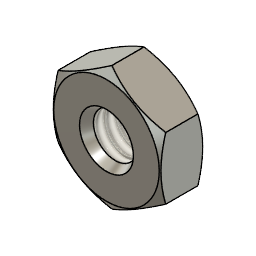
Gimbal Mechanism - Model Rocketry (Autodesk Fusion 360 archive; units mm, degrees)
design "Hexagon Regular Nut ISO 4032 - M2 Steel 6 Plain"
description: Hexagon Regular Nut ISO 4032 - M2
part number: ISO 4032 - M2 Steel 6 Plain
Autodesk Fusion 360 part; units mm, degrees
sketch "Sketch1" plane through (0, 0, 0) normal (0, 1, 0) x (1, 0, 0)
  line L0 (0, 0) -> (0, -1.6)
  line L1 (-1, 0) -> (-1.96, 0)
  line L2 (-1.96, 0) -> (-2.31, -0.2021)
  line L3 (-2.31, -0.2021) -> (-2.31, -1.3979)
  line L4 (-2.31, -1.3979) -> (-1.96, -1.6)
  line L5 (-1.96, -1.6) -> (-1, -1.6)
  line L6 (-1, -1.6) -> (-1, 0)
  dimension "d121" = 2
  dimension "d122" = 30
  dimension "d123" = 30
  dimension "d128" = 4.62
  dimension "d172" = 3.92
  dimension "d179" = 1.6
  constraint vertical L0
  constraint coincident L0 L0.end
  constraint coincident origin L0
  constraint horizontal L1
  constraint coincident L0.start L1
  constraint coincident L0.start origin
  constraint coincident L0.end L5
  constraint vertical L1.end L4.end
  measures "d122" angle of L1 L2
  measures "d123" angle of L4 L5
  measures "d179" distance of L1 L5
revolve "Revolve1" add sketch "Sketch1" angle 360 about axis through (0, 0, 0) along (0, 0, 1)
sketch "Sketch8" plane through (0, 0, 1.6) normal (0, 0, 1) x (1, 0, 0)
  line L0 (-2, -1.1559) -> (-2, 1.1559)
  circle A0 centre (0, 0) radius 1
  circle A1 centre (0, 0) radius 2.31
  dimension "d114" = 2
  constraint coincident L0.end A1
  constraint coincident L0.start A1
  constraint vertical L0
  measures "d114" distance of A0.centre L0
extrude "Extrude5" cut sketch "Sketch8" against normal blind 1.6 contours L0 A1 picked at (-2.05, 0.2815)
pattern_circular "C-Pattern2" count 6 over 360 about axis through (0, 0, 1.75) along (0, 0, 1) of "Extrude5"
thread "Thread3" "ISO Metric profile 2.0 M2x0.4 M2x0.4 6H" major diameter 2.074 minor diameter 1.623 pitch 0.4 angle 60 resizes the face on face at (-0.9988, 0.0498, 1.0667)
sketch "Sketch12" plane through (0, 0, 0) normal (0, 1, 0) x (1, 0, 0)
  line L0 (-1, 0) -> (0, 0)
  line L1 (-0.5381, -0.8) -> (-1, 0)
  line L2 (-1, -1.6) -> (0, -1.6)
  line L3 (-0.5381, -0.8) -> (-1, -1.6)
  line L4 (0, 0) -> (0, -1.6)
  dimension "d169" = 60
  dimension "d177" = 1
  dimension "d178" = 60
  constraint horizontal L0
  constraint coincident L1.start L3.start
  constraint vertical L0.start L2.start
  constraint coincident L2.end L4.end
  constraint coincident L0.end L4.start
  constraint perpendicular L2 L4
  measures "d169" angle of L2 L3
  measures "d177" distance of L0.start L4
  measures "d178" angle of L0 L1
revolve "Revolve3" cut sketch "Sketch12" angle 360 about axis through (0, 0, 1.75) along (0, 0, 1)
equation "adsk_nheig = 1.60 mm"
equation "adsk_maxdia = 4.62 mm"
equation "adsk_nomdia = 2.00 mm"
equation "d89 = -adsk_nheig"
equation "adsk_waflat = 4.00 mm"
equation "d114 = adsk_waflat / 2"
equation "adsk_chamang1 = 30.00 deg"
equation "adsk_chamang2 = 30.00 deg"
equation "d121 = adsk_nomdia"
equation "d122 = adsk_chamang1"
equation "d123 = adsk_chamang2"
equation "d128 = adsk_maxdia"
equation "d163 = adsk_nheig"
equation "adsk_beardia = 3.92 mm"
equation "d172 = adsk_beardia"
equation "d177 = adsk_nomdia * 0.5"
equation "d179 = adsk_nheig"

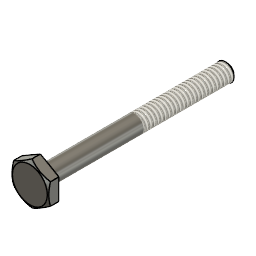
design "Hexagon Head Bolt ISO 4014 - M2 x 20 Steel 4.6 Plain"
description: Hexagon Head Bolt ISO 4014 - M2 x 20
part number: ISO 4014 - M2 x 20 Steel 4.6 Plain
Autodesk Fusion 360 part; units mm, degrees
sketch "Sketch1" plane through (0, 0, 0) normal (0, 1, 0) x (1, 0, 0)
  line L0 (-1, 0) -> (-1, 20)
  line L1 (-1, 20) -> (0, 20)
  line L2 (0, 20) -> (0, -1.4)
  line L3 (-1.67, -0.25) -> (-2.31, -0.25)
  line L4 (-2.31, -0.25) -> (-2.31, -1.1633)
  line L5 (-1.67, -0.25) -> (-1.5257, 0)
  line L6 (-1.5257, 0) -> (-1, 0)
  line L7 (0, -1.4) -> (-1.9, -1.4)
  line L8 (-2.31, -1.1633) -> (-1.9, -1.4)
  dimension "d81" = 4.62
  dimension "d123" = 0.25
  dimension "d127" = 20
  dimension "d149" = 2
  dimension "d157" = 30
  dimension "d158" = 3.8
  dimension "d162" = 1.4
  dimension "d163" = 30
  dimension "d164" = 3.34
  constraint perpendicular L0 L1
  constraint vertical L2
  constraint parallel L2 L4
  constraint coincident L2 L7.start
  constraint coincident origin L6
  constraint coincident L0.end L1.start
  constraint perpendicular L2 L7
  constraint coincident origin L2
  measures "d123" distance of L3 L6
  measures "d127" distance of L1 L6
  measures "d157" angle of L7 L8
  measures "d162" distance of L6 L7
  measures "d163" angle of L4 L5
revolve "Revolve1" add sketch "Sketch1" angle 360 about axis through (0, 0, -20) along (0, 0, 1)
sketch "Sketch8" plane through (0, 0, 0) normal (0, 0, 1) x (1, 0, 0)
  circle A0 centre (0, 0) radius 2.31
  circle A1 centre (0, 0) radius 2.31
  line L0 (-2.0005, -1.155) -> (0, -2.31)
  line L1 (0, -2.31) -> (2.0005, -1.155)
  line L2 (2.0005, -1.155) -> (2.0005, 1.155)
  line L3 (2.0005, 1.155) -> (0, 2.31)
  line L4 (0, 2.31) -> (-2.0005, 1.155)
  line L5 (-2.0005, 1.155) -> (-2.0005, -1.155)
  constraint coincident A1 L0.start
  constraint coincident A0.centre A1.centre
  constraint vertical L5
extrude "Extrude5" cut sketch "Sketch8" along normal through all contours A0 A1 L2 | A0 A1 L3 | A0 A1 L1 | A0 A1 L4 | A0 A1 L0 | A0 A1 L5
thread "Thread2" "ISO Metric profile 2.0 M2x0.4 M2x0.4 6g" major diameter 1.9335 minor diameter 1.478 pitch 0.4 angle 60 resizes the face on face at (-0.995, 0.0996, -13.3333) from (0, 0, -10) to (0, 0, -20)
fillet "Fillet6" radius 0.1 1 edges at (0.9668, 0, 0)
sketch "Sketch15" plane through (0, 0, 0) normal (0, 1, 0) x (1, 0, 0)
  line L0 (-1.02, 20) -> (-1.02, 19.7546)
  line L1 (-1.02, 19.7546) -> (-0.7546, 20)
  line L2 (0, 20) -> (0, -1.4)
  line L3 (-1.02, 20) -> (0, 20)
  dimension "d165" = 0.7546
  dimension "d166" = 1.02
  dimension "d167" = 0.2454
  constraint coincident L2.start L3.end
  constraint perpendicular L2 L3
  constraint coincident L1.end L3
  constraint perpendicular L0 L3
  measures "d165" distance of L1.end L2
  measures "d166" distance of L0 L2.start
  measures "d167" distance of L0.end L3
revolve "Revolve4" cut sketch "Sketch15" angle 360 about axis through (0, 0, 1.75) along (0, 0, 1)
equation "adsk_nomlen = 20.00 mm"
equation "adsk_headh = 1.40 mm"
equation "adsk_headdia = 4.62 mm"
equation "adsk_nomdia = 2.00 mm"
equation "d81 = adsk_headdia"
equation "adsk_waflat = 4.00 mm"
equation "adsk_thrlen = 10.00 mm"
equation "adsk_chamang2 = 30.00 deg"
equation "adsk_midfillet = 0.10 mm"
equation "d123 = adsk_necklen"
equation "adsk_necklen = 0.25 mm"
equation "adsk_neckdia = 3.34 mm"
equation "d127 = adsk_nomlen"
equation "d138 = adsk_midfillet"
equation "d140 = min(adsk_thrlen; adsk_nomlen - adsk_midfillet - 0.01 mm)"
equation "adsk_endpointdia = 1.50924 mm"
equation "adsk_startlen = 0.24538 mm"
equation "d149 = adsk_nomdia"
equation "d157 = adsk_chamang2"
equation "d158 = adsk_waflat * 0.95"
equation "adsk_neckang = 30 deg"
equation "d162 = adsk_headh"
equation "d163 = adsk_neckang"
equation "d164 = adsk_neckdia"
equation "d165 = adsk_endpointdia / 2"
equation "d166 = adsk_nomdia * 0.51"
equation "d167 = adsk_startlen"
